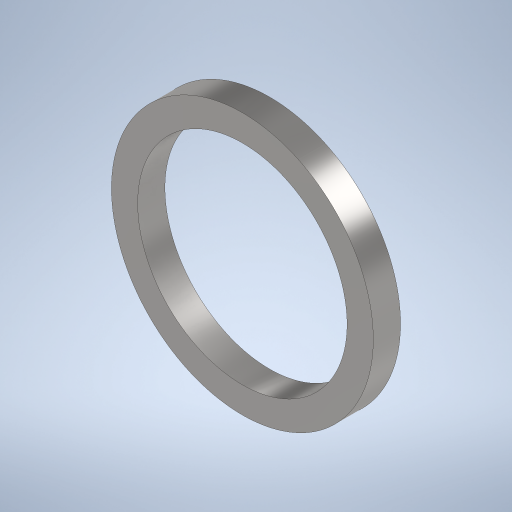
# Autodesk Inventor part: 6820ZZ
Saved by Autodesk Inventor 2024 (Build 280153000, 153)
## iProperties
Created: 2023-05-29
Part Number: 6820ZZ
Material: 鋼、炭素鋼
Document SubType Name: Modeling
Designer: yuta2
Density: 5.22355 g/cm^3
Appearance: 半つや出し
Mass: 300 g
Surface Area: 180.249 cm^2
Volume: 57.4322 cm^3
Author: yuta2
Autodesk Inventor part; units mm, degrees
ref_plane "YZ Plane" through (0, 0, 0) normal (1, 0, 0) x (0, 1, 0)
ref_plane "XZ Plane" through (0, 0, 0) normal (0, 1, 0) x (-1, 0, 0)
ref_plane "XY Plane" through (0, 0, 0) normal (0, 0, 1) x (1, 0, 0)
sketch "スケッチ1" plane through (0, 0, 0) normal (0, 0, 1) x (1, 0, 0)
  circle A0 centre (0, 0) radius 50
  circle A1 centre (0, 0) radius 62.5
  dimension "d0" = 100
  dimension "d1" = 125
  constraints: 2 centre point, 2 coincident
  measures "d0" diameter of A0
  measures "d1" diameter of A1
extrude "押し出し1" add sketch "スケッチ1" along normal blind 13
